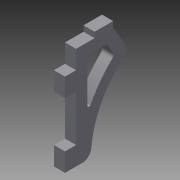
# Autodesk Inventor part: HarnessPusher27021014
Saved by Autodesk Inventor 2015 (Build 190159000, 159)
## iProperties
Created: 2014-07-21
Part Number: HarnessPusher27021014
Material: Generic
Document SubType Name: Modeling
Designer: STACKPOLE
Density: 1 g/cm^3
Appearance: Default
Author: STACKPOLE
Autodesk Inventor part; units mm, degrees
ref_plane "YZ Plane" through (0, 0, 0) normal (1, 0, 0) x (0, 1, 0)
ref_plane "XZ Plane" through (0, 0, 0) normal (0, 1, 0) x (-1, 0, 0)
ref_plane "XY Plane" through (0, 0, 0) normal (0, 0, 1) x (1, 0, 0)
sketch "Sketch1" plane through (0, 0, 0) normal (1, 0, 0) x (0, 1, 0)
  line L0 (-29.5376, 40.3427) -> (-38, 55)
  circle A0 centre (0, 0) radius 50 construction
  line L1 (-38, 55) -> (-38.0101, 58)
  line L2 (-38.0101, 58) -> (-48.0101, 58)
  line L3 (-48.0101, 58) -> (-48, 55)
  line L4 (-58, 35) -> (-64, 35)
  line L5 (-64, 35) -> (-64, 45)
  line L6 (-64, 45) -> (-58, 45)
  arc A1 (-42.0654, 27.0278) -> (-29.5376, 40.3427) centre (0, 0) ccw construction
  line L7 (-58, 55) -> (-58, 45)
  line L8 (-38, 55) -> (-38, 55)
  line L9 (-48, 55) -> (-58, 55)
  line L10 (-58, 55) -> (-36.8235, 33.8235) construction
  line L11 (-50, 0) -> (-57.2434, 0)
  line L12 (-57.2434, 0) -> (-64, 0)
  line L13 (-64, 0) -> (-64, 10)
  line L14 (-64, 10) -> (-58, 10)
  line L15 (-58, 35) -> (-58, 10)
  arc A2 (-29.5376, 40.3427) -> (-50, 0) centre (0, 0) ccw
  point P0 (-30.8961, 39.312)
  dimension "d6" = 50
  dimension "d8" = 10
  dimension "d10" = 3
  dimension "d11" = 10
  dimension "d12" = 6
  dimension "d17" = 120
  dimension "d18" = 10
  dimension "d19" = 5
  dimension "d21" = 10
  dimension "d23" = 45
  dimension "d25" = 15
  dimension "d26" = 0
  dimension "d30" = 10
  dimension "d31" = 6
  dimension "d32" = 25
  dimension "d38" = 58
  constraints: 33 end point, 11 point on circle, 4 parallel, 3 centre point, 3 horizontal, 2 coincident, 2 perpendicular, 2 vertical, 1 horizontal alignment, 1 vertical alignment
  measures "d6" radius of A0
  measures "d8" distance of L1.end L2.end
  measures "d10" distance of L2.end L3.end
  measures "d11" distance of L4.end L5.end
  measures "d12" distance of L4.start L4.end
  measures "d17" angle of L0 L8
  measures "d18" distance of L3.end L7.start
  measures "d19" distance edge to line of A1 L8
  measures "d21" distance between parallel lines of L6 L9
  measures "d23" angle of L9 L10
  measures "d25" angle of L10 L0
  measures "d26" distance of L0.end L1.start
  measures "d30" distance of L12.end L13.end
  measures "d31" distance of L14.end L13.end
  measures "d32" distance of L4.start L14.end
  measures "d38" distance from line of L15 A0.centre
extrude "Extrusion2" add sketch "Sketch1" along normal blind 6
fillet "Fillet3" radius 5 2 edges at (3, -29.5376, 40.3427) (3, -50, 0)
sketch "Sketch2" plane through (6, 0, 0) normal (1, 0, 0) x (0, 0, -1)
  arc A0 (-41.7758, -37.2932) -> (-20.7846, -52) centre (0, 0) ccw
  line L0 (-20.7846, -52) -> (-49, -52)
  line L1 (-49, -52) -> (-49, -41.4641)
  line L2 (-49, -41.4641) -> (-41.7758, -37.2932)
  line L3 (-44.0661, -31.6873) -> (-55, -38) projected
  line L4 (-55, -48) -> (-55, -58) projected
  line L5 (-55, -58) -> (-45, -58) projected
  dimension "d42" = 6
  dimension "d43" = 6
  dimension "d44" = 6
  dimension "d45" = 56
  constraints: 6 end point, 3 parallel, 2 point on circle, 1 centre point, 1 coincident, 1 horizontal, 1 perpendicular
  measures "d42" distance between parallel lines of L5 L0
  measures "d43" distance between parallel lines of L4 L1
  measures "d44" distance between parallel lines of L3 L2
  measures "d45" radius of A0
extrude "Extrusion3" cut sketch "Sketch2" against normal through all
fillet "Fillet4" radius 1 1 edges at (3, -52, 20.7846)
fillet "Fillet5" radius 2 3 edges at (3, -52, 49) (3, -41.4641, 49) (3, -37.2932, 41.7758)
body "Solid2"
